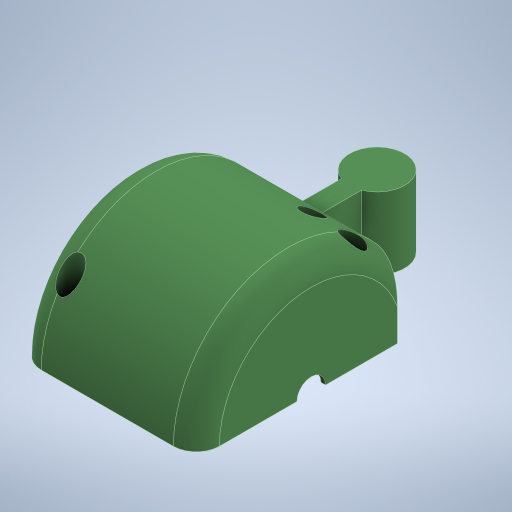
# Autodesk Inventor part: Arm_1Up
Saved by Autodesk Inventor 2023 (Build 270158000, 158)
## iProperties
Created: 2024-07-29
Part Number: Arm_1Up
Material: Generic
Document SubType Name: Modeling
Designer: Swoby
Density: 1 g/cm^3
Appearance: Default
Author: Swoby
Autodesk Inventor part; units mm, degrees
ref_plane "YZ Plane" through (0, 0, 0) normal (1, 0, 0) x (0, 1, 0)
ref_plane "XZ Plane" through (0, 0, 0) normal (0, 1, 0) x (-1, 0, 0)
ref_plane "XY Plane" through (0, 0, 0) normal (0, 0, 1) x (1, 0, 0)
sketch "Sketch1" plane through (0, 0, 0) normal (1, 0, 0) x (0, 1, 0)
  arc A0 (26.4575, -30) -> (0, 40) centre (0, 0) ccw
  line L0 (0, 40) -> (0, -30)
  line L1 (0, -30) -> (26.4575, -30)
  arc A1 (0, 40) -> (26.4575, -30) centre (0, 0) ccw construction
  dimension "d0" = 80
  dimension "d1" = 70
  constraints: 4 end point, 4 point on circle, 2 centre point, 1 coincident, 1 perpendicular, 1 point on line, 1 vertical
  measures "d0" diameter of A0
  measures "d1" distance from line of L0.start L1
extrude "Extrusion1" add sketch "Sketch1" along normal blind 62
fillet "Fillet1" radius 8 2 edges at (0, 37.4166, 14.1421) (62, 37.4166, 14.1421)
sketch "Sketch2" plane through (0, 0, -30) normal (0, -1, 0) x (1, 0, 0)
  circle A0 centre (31, -23.9392) radius 9.6
  line L0 (0, 0) -> (62, 0) projected
  line L1 (31, -23.9392) -> (31, 0) construction
  line L2 (34.5, 0) -> (27.5, 0)
  line L3 (27.5, 0) -> (27.5, -15)
  line L4 (34.5, 0) -> (34.5, -15)
  point P0 (0, 30)
  dimension "d6" = 19.2
  dimension "d7" = 3.5
  dimension "d8" = 3.5
  dimension "d61" = 15
  constraints: 8 end point, 3 point on line, 2 midpoint, 2 parallel, 2 point on circle, 1 centre point, 1 perpendicular
  measures "d6" diameter of A0
  measures "d7" distance between parallel lines of L4 L1
  measures "d8" distance between parallel lines of L3 L1
  measures "d61" distance of L2.end L3.end
extrude "Extrusion2" add sketch "Sketch2" against normal blind 25
sketch "Sketch3" plane through (34.5, 0, -30) normal (1, 0, 0) x (0, 0, -1)
  line L0 (0, 25) -> (15, 25) projected
  line L1 (0, 11.1355) -> (0, 26.4575) projected
  arc A0 (1.225, 25) -> (0, 26.4575) centre (-30.0052, -0.0046) ccw
  arc A1 (0, 26.4575) -> (-70, 0) centre (-30, 0) ccw projected
  line L2 (0, 26.4575) -> (1.225, 25) construction
  point P0 (-30, 0)
  dimension "d13" = 1.225
  constraints: 2 end point, 2 point on circle, 1 centre point, 1 point on line, 1 tangent
  measures "d13" distance from line of L1 L2.end
extrude "Extrusion3" add sketch "Sketch3" against normal up to surface (7 mm away)
sketch "Sketch4" plane through (0, 0, -30) normal (0, -1, 0) x (1, 0, 0)
  line L0 (58.9, 60.95) -> (51.4, 60.95)
  line L1 (18.3, 60.95) -> (18.3, 19.35)
  line L2 (58.9, 19.35) -> (58.9, 60.95)
  line L3 (58.9, 37.4) -> (60.4, 37.4)
  line L4 (60.4, 37.4) -> (60.4, 30)
  line L5 (60.4, 22.6) -> (58.9, 22.6)
  line L6 (58.9, 22.6) -> (58.9, 37.4)
  line L7 (60.4, 35) -> (62, 35)
  line L8 (62, 35) -> (62, 30)
  line L9 (62, 25) -> (60.4, 25)
  line L10 (60.4, 25) -> (60.4, 35)
  line L11 (47.7, 19.35) -> (47.7, 12.25)
  line L12 (47.7, 12.25) -> (51.4, 12.25)
  line L13 (51.4, 12.25) -> (51.4, 19.35)
  line L14 (22.2, 19.35) -> (22.2, 13.35)
  line L15 (22.2, 13.35) -> (27.6, 13.35)
  line L16 (27.6, 13.35) -> (27.6, 19.35)
  line L17 (47.7, 60.95) -> (47.7, 68.05)
  line L18 (47.7, 68.05) -> (51.4, 68.05)
  line L19 (51.4, 68.05) -> (51.4, 60.95)
  line L20 (47.7, 60.95) -> (18.3, 60.95)
  line L21 (51.4, 19.35) -> (58.9, 19.35)
  line L22 (18.3, 19.35) -> (22.2, 19.35)
  line L23 (27.6, 19.35) -> (47.7, 19.35)
  line L24 (62, 62) -> (62, 0) projected
  line L25 (54, 0) -> (54, 70) projected
  line L26 (0, 30) -> (48.0104, 30) construction
  line L27 (62, 30) -> (58.9, 30)
  line L28 (62, 30) -> (62, 25)
  line L29 (60.4, 30) -> (60.4, 22.6)
  dimension "d16" = 40.6
  dimension "d17" = 41.6
  dimension "d18" = 10
  dimension "d19" = 14.8
  dimension "d20" = 1.6
  dimension "d21" = 1.5
  dimension "d22" = 10.65
  dimension "d23" = 3.7
  dimension "d24" = 7.5
  dimension "d25" = 7.1
  dimension "d26" = 7.1
  dimension "d27" = 3.9
  dimension "d28" = 5.4
  dimension "d29" = 6
  dimension "d30" = 5
  constraints: 56 end point, 18 parallel, 10 perpendicular, 6 point on line, 5 collinear, 5 horizontal, 1 midpoint
  measures "d16" distance between parallel lines of L1 L2
  measures "d17" distance of L2.start L0.start
  measures "d18" distance of L7.end L9.start
  measures "d19" distance of L3.end L5.start
  measures "d20" distance of L9.start L9.end
  measures "d21" distance of L5.start L5.end
  measures "d22" distance between parallel lines of L23 L26
  measures "d23" distance of L11.end L12.end
  measures "d24" distance of L13.end L2.start
  measures "d25" distance of L12.end L13.end
  measures "d26" distance of L18.end L0.end
  measures "d27" distance of L1.end L14.start
  measures "d28" distance of L14.end L15.end
  measures "d29" distance of L15.end L16.end
  measures "d30" distance between parallel lines of L9 L27
extrude "Extrusion4" cut sketch "Sketch4" against normal blind 10.6 contours L2 L21 L25 L0 | L25 L21 L13 L12 L11 L23 L16 L15 L14 L22 L1 L20 L17 L18 L19 L0
revolve "Revolution1" cut sketch "Sketch4" angle 360 about axis through (62, 0, 0) along (-1, 0, 0) contours L27 L10 L29 L5 L2 | L27 L24 L9 L10
sketch "Sketch5" plane through (0, 0, -30) normal (0, -1, 0) x (1, 0, 0)
  line L0 (0, 30) -> (14.3, 30)
  line L1 (14.3, 30) -> (14.3, 17.6)
  line L2 (14.3, 17.6) -> (0, 17.6)
  line L3 (0, 17.6) -> (0, 30)
  dimension "d34" = 24.8
  dimension "d35" = 14.3
  constraints: 8 end point, 3 perpendicular, 1 horizontal
  measures "d34" diameter of L2 L0
  measures "d35" distance of L1.end L2.end
revolve "Revolution2" cut sketch "Sketch5" angle 360 about axis through (0, 0, 0) along (1, 0, 0)
sketch "Sketch6" plane through (8, 0, 40) normal (0, -1, 0) x (1, 0, 0)
  line L0 (6.3, -52.4) -> (-8, -52.4) projected
  line L1 (6.3, -27.6) -> (6.3, -52.4) projected
  line L2 (-8, -27.6) -> (6.3, -27.6) projected
  line L3 (-8, -52.4) -> (-8, -27.6) projected
  line L4 (6.3, -52.4) -> (-3, -52.4)
  line L5 (-3, -52.4) -> (-3, -65.75)
  line L6 (-3, -65.75) -> (6.3, -65.75)
  line L7 (6.3, -65.75) -> (6.3, -52.4)
  line L8 (-8, -70) -> (19.5, -70) projected
  line L9 (-3, -52.4) -> (6.3, -52.4)
  line L10 (6.3, -52.4) -> (6.3, -40)
  line L11 (6.3, -40) -> (-3, -40)
  line L12 (-3, -40) -> (-3, -52.4)
  point P0 (-8, -40)
  dimension "d38" = 5
  dimension "d39" = 4.25
  constraints: 16 end point, 4 parallel, 2 horizontal, 2 perpendicular, 1 midpoint
  measures "d38" distance between parallel lines of L3 L5
  measures "d39" distance between parallel lines of L8 L6
extrude "Extrusion5" cut sketch "Sketch6" against normal blind 12.4 contours L7 L6 L5 L0 | L0 L12 L11 L1
sketch "Sketch7" plane through (8, 0, 40) normal (0, -1, 0) x (1, 0, 0)
  line L0 (-3, -65.75) -> (-3, -52.4) projected
  line L1 (-3, -52.4) -> (-8, -52.4) projected
  line L2 (-8, -52.4) -> (-8, -70) projected
  line L3 (-8, -70) -> (19.5, -70) projected
  line L4 (19.5, -70) -> (19.5, -85) projected
  arc A0 (19.5, -85) -> (26.5, -85) centre (23, -93.9392) ccw projected
  line L5 (26.5, -85) -> (26.5, -70) projected
  line L6 (26.5, -70) -> (54, -70) projected
  line L7 (54, -45) -> (54, -70) projected
  line L8 (54, -45) -> (52.4, -45) projected
  line L9 (52.4, -45) -> (52.4, -47.4) projected
  line L10 (52.4, -47.4) -> (50.9, -47.4) projected
  line L11 (50.9, -47.4) -> (50.9, -50.65) projected
  line L12 (50.9, -50.65) -> (43.4, -50.65) projected
  line L13 (43.4, -50.65) -> (43.4, -57.75) projected
  line L14 (43.4, -57.75) -> (39.7, -57.75) projected
  line L15 (39.7, -57.75) -> (39.7, -50.65) projected
  line L16 (39.7, -50.65) -> (19.6, -50.65) projected
  line L17 (19.6, -50.65) -> (19.6, -56.65) projected
  line L18 (19.6, -56.65) -> (14.2, -56.65) projected
  line L19 (14.2, -56.65) -> (14.2, -50.65) projected
  line L20 (14.2, -50.65) -> (10.3, -50.65) projected
  line L21 (10.3, -50.65) -> (10.3, -9.05) projected
  line L22 (10.3, -9.05) -> (39.7, -9.05) projected
  line L23 (39.7, -9.05) -> (39.7, -1.95) projected
  line L24 (39.7, -1.95) -> (43.4, -1.95) projected
  line L25 (43.4, -1.95) -> (43.4, -9.05) projected
  line L26 (43.4, -9.05) -> (50.9, -9.05) projected
  line L27 (50.9, -9.05) -> (50.9, -32.6) projected
  line L28 (50.9, -32.6) -> (52.4, -32.6) projected
  line L29 (52.4, -32.6) -> (52.4, -35) projected
  line L30 (52.4, -35) -> (54, -35) projected
  line L31 (54, -8) -> (54, -35) projected
  arc A1 (54, -8) -> (46, 0) centre (46, -8) ccw projected
  line L32 (0, 0) -> (46, 0) projected
  arc A2 (0, 0) -> (-8, -8) centre (0, -8) ccw projected
  line L33 (-8, -8) -> (-8, -27.6) projected
  line L34 (-8, -27.6) -> (6.3, -27.6) projected
  line L35 (6.3, -27.6) -> (6.3, -65.75) projected
  line L36 (6.3, -65.75) -> (-3, -65.75) projected
  circle A3 centre (1.15, -9.15) radius 2
  circle A4 centre (34, -60.325) radius 2
  circle A5 centre (48, -60.325) radius 2
  point P0 (-8, -40)
  dimension "d42" = 4
  dimension "d43" = 4
  dimension "d44" = 18.3
  dimension "d45" = 9.15
  dimension "d46" = 9.15
  dimension "d47" = 19.35
  dimension "d48" = 9.675
  dimension "d49" = 20
  dimension "d52" = 4
  dimension "d53" = 6
  dimension "d54" = 9.675
  constraints: 3 centre point
  measures "d42" diameter of A3
  measures "d43" diameter of A4
  measures "d44" distance between parallel lines of L33 L21
  measures "d45" distance from line of L33 A3.centre
  measures "d46" distance from line of L32 A3.centre
  measures "d47" distance between parallel lines of L6 L12
  measures "d48" distance from line of L6 A4.centre
  measures "d49" distance from line of L7 A4.centre
  measures "d52" diameter of A5
  measures "d53" distance from line of L7 A5.centre
  measures "d54" distance from line of L6 A5.centre
extrude "Extrusion6" cut sketch "Sketch7" against normal through all contours A3 | A4 | A5
ref_plane "Work Plane1" through (8, 6, 40) normal (0, -1, 0) x (1, 0, 0)
sketch "Sketch8" plane through (8, 6, 40) normal (0, -1, 0) x (1, 0, 0)
  circle A0 centre (48, -60.325) radius 2 projected
  circle A1 centre (34, -60.325) radius 2 projected
  circle A2 centre (1.15, -9.15) radius 2 projected
  circle A3 centre (1.15, -9.15) radius 3.75
  circle A4 centre (34, -60.325) radius 3.75
  circle A5 centre (48, -60.325) radius 3.75
  point P0 (-8, -40)
  dimension "d56" = 7.5
  dimension "d57" = 7.5
  dimension "d58" = 7.5
  constraints: 3 centre point, 3 coincident
  measures "d56" diameter of A3
  measures "d57" diameter of A4
  measures "d58" diameter of A5
extrude "Extrusion7" cut sketch "Sketch8" against normal through all contours A0 | A1 | A2 | A3 | A4 | A5
sketch "Sketch9" plane through (34.5, 0, -30) normal (1, 0, 0) x (0, 0, -1)
  circle A0 centre (9.225, 12.5) radius 2
  line L0 (1.225, 25) -> (15, 25) projected
  line L1 (15, 0) -> (15, 25) projected
  line L2 (0, 0) -> (0, 11.1355) projected
  point P0 (-30, 0)
  point P1 (8.1125, 25)
  dimension "d62" = 4
  dimension "d63" = 12.5
  dimension "d67" = 9.225
  constraints: 1 centre point, 1 midpoint
  measures "d62" diameter of A0
  measures "d63" vertical distance of A0.centre point (8.113, 25)
  measures "d67" distance from line of L2 A0.centre
extrude "Extrusion8" cut sketch "Sketch9" against normal through all
equation "\"d26\" = d25"
equation "\"d45\" = 0.5 * d44"
equation "\"d46\" = d45"
equation "\"d48\" = 0.5 * d47"
equation "\"d54\" = d48"
body "Solid1"
